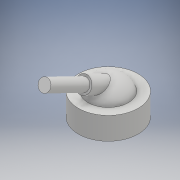
# Autodesk Inventor part: waterbottle_lid
Saved by Autodesk Inventor 2017.2 (Build 212233000, 233)
## iProperties
Created: 2017-08-24
Part Number: waterbottle_lid
Material: Generic
Document SubType Name: Modeling
Designer: Nic
Density: 1 g/cm^3
Appearance: Default
Author: Nic
Autodesk Inventor part; units mm, degrees
ref_plane "YZ Plane" through (0, 0, 0) normal (1, 0, 0) x (0, 1, 0)
ref_plane "XZ Plane" through (0, 0, 0) normal (0, 1, 0) x (-1, 0, 0)
ref_plane "XY Plane" through (0, 0, 0) normal (0, 0, 1) x (1, 0, 0)
sketch "Sketch1" plane through (0, 0, 0) normal (0, 1, 0) x (-1, 0, 0)
  line L0 (0, 0) -> (20, 0)
  line L1 (20, 0) -> (20, 15)
  line L2 (20, 15) -> (13.5, 15)
  line L3 (0, 25) -> (0, 0)
  line L4 (0, 0) -> (0, 15.843) construction
  line L5 (0, 25) -> (13.5, 25) construction
  line L6 (13.5, 25) -> (13.5, 15) construction
  line L7 (0, 0) -> (0, -31.0844) construction
  arc A0 (13.5, 15) -> (0, 25) centre (0, 10.8875) ccw
  dimension "d0" = 20
  dimension "d1" = 15
  dimension "d3" = 25
  dimension "d4" = 13.5
  constraints: 16 end point, 3 perpendicular, 3 vertical, 2 horizontal, 2 point on circle, 2 point on line, 1 centre point
  measures "d0" distance of L0.start L0.end
  measures "d1" distance of L0.end L1.end
  measures "d3" distance between parallel lines of L0 L5
  measures "d4" distance of L3.start L5.end
revolve "Revolution1" add sketch "Sketch1" angle 360 about axis through (0, 0, 0) along (0, 0, -1)
sketch "Sketch2" plane through (0, 0, 0) normal (1, 0, 0) x (0, 1, 0)
  line L0 (0, 19) -> (-45.3208, 41.1044) construction
  line L1 (0, 19) -> (-38.3392, 19) construction
  line L2 (-20, 0) -> (20, 0) construction
  line L3 (0, 19) -> (0, 0) construction
  line L4 (0, 19) -> (2.3014, 23.7187)
  line L5 (2.3014, 23.7187) -> (-14.3262, 31.8285)
  line L6 (-14.3262, 31.8285) -> (-14.8742, 30.705)
  line L7 (-14.8742, 30.705) -> (-40.9392, 43.4178)
  line L8 (-40.9392, 43.4178) -> (-42.6927, 39.8226)
  line L9 (-42.6927, 39.8226) -> (0, 19)
  dimension "d6" = 19
  dimension "d7" = 26
  dimension "d8" = 18.5
  dimension "d9" = 29
  dimension "d10" = 4
  dimension "d11" = 5.25
  constraints: 18 end point, 4 perpendicular, 1 collinear, 1 horizontal, 1 vertical
  measures "d6" distance between parallel lines of L2 L1
  measures "d7" angle of L0 L1
  measures "d8" distance of L4.end L5.end
  measures "d9" distance between parallel lines of L6 L8
  measures "d10" distance of L7.end L8.end
  measures "d11" distance between parallel lines of L0 L5
revolve "Revolution2" add sketch "Sketch2" angle 360 about axis through (0, 0, 19) along (0, -0.898794, 0.4383711)
sketch "Sketch3" plane through (0, 0, 0) normal (0, 0, -1) x (-1, 0, 0)
  circle A0 centre (0, 0) radius 9.1875
  dimension "d13" = 18.375
  constraints: 1 centre point, 1 coincident
  measures "d13" diameter of A0
extrude "Extrusion1" cut sketch "Sketch3" against normal blind 12
body "Solid1"
